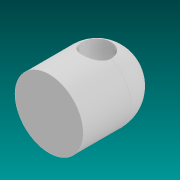
# Autodesk Inventor part: bevestiging axis 2
Saved by Autodesk Inventor 2020.2 (Build 242310000, 310)
## iProperties
Created: 2020-05-18
Part Number: bevestiging axis 2
Material: Generic
Document SubType Name: Modeling
Designer: Svend
Density: 1 g/cm^3
Appearance: Default
Author: Svend
Autodesk Inventor part; units mm, degrees
ref_plane "YZ Plane" through (0, 0, 0) normal (1, 0, 0) x (0, 1, 0)
ref_plane "XZ Plane" through (0, 0, 0) normal (0, 1, 0) x (-1, 0, 0)
ref_plane "XY Plane" through (0, 0, 0) normal (0, 0, 1) x (1, 0, 0)
sketch "Sketch1" plane through (0, 0, 0) normal (0, 0, 1) x (1, 0, 0)
  circle A0 centre (0, 0) radius 50
  dimension "d0" = 100
  constraints: 1 centre point, 1 coincident
  measures "d0" diameter of A0
extrude "Extrusion1" add sketch "Sketch1" along normal blind 10
sketch "Sketch2" plane through (0, 0, 0) normal (0, 1, 0) x (-1, 0, 0)
  circle A0 centre (0, -60) radius 21
  circle A1 centre (0, -60) radius 50
  line L0 (50, 0) -> (-50, 0) projected
  line L1 (50, -60) -> (50, 0)
  line L2 (-50, -60) -> (-50, 0)
  line L3 (0, -110) -> (0, 0)
  dimension "d3" = 42
  dimension "d4" = 100
  dimension "d5" = 60
  constraints: 6 end point, 3 point on circle, 3 vertical, 2 centre point, 1 coincident, 1 vertical alignment
  measures "d3" diameter of A0
  measures "d4" diameter of A1
  measures "d5" distance from line of L0 A1.centre
revolve "Revolution1" add sketch "Sketch2" angle 360 about axis through (0, 0, -110) along (0, 0, 1) picked at (-4.9283, -53.5984) picked at (-35.0167, -40.386) contours L3 A0 | A0 L3 A1 | A1 L2 L0 L3
sketch "Sketch3" plane through (0, 0, 0) normal (0, 1, 0) x (-1, 0, 0)
  circle A0 centre (0, -60) radius 21
  arc A1 (-50, -60) -> (50, -60) centre (0, -60) ccw projected
  point P0 (0, 0)
  dimension "d7" = 42
  constraints: 1 centre point, 1 coincident
  measures "d7" diameter of A0
extrude "Extrusion2" cut sketch "Sketch3" along normal through all both and the other way through all
body "Solid1"
